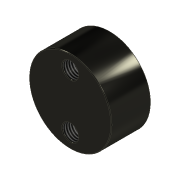
# Autodesk Inventor part: draaischijf HMI
Saved by Autodesk Inventor 2020.3 (Build 243373000, 373)
## iProperties
Created: 2020-12-03
Part Number: draaischijf HMI
Material: Stainless Steel
Document SubType Name: Modeling
Designer: Svend
Density: 8 g/cm^3
Appearance: Gunmetal
Author: Svend
Autodesk Inventor part; units mm, degrees
ref_plane "YZ Plane" through (0, 0, 0) normal (1, 0, 0) x (0, 1, 0)
ref_plane "XZ Plane" through (0, 0, 0) normal (0, 1, 0) x (-1, 0, 0)
ref_plane "XY Plane" through (0, 0, 0) normal (0, 0, 1) x (1, 0, 0)
sketch "Sketch1" plane through (0, 0, 0) normal (0, 0, 1) x (1, 0, 0)
  circle A0 centre (0, 0) radius 13
  circle A1 centre (0, 8.5) radius 2.5
  circle A2 centre (0, -8.5) radius 2.5
  line L0 (0, 8.5) -> (0, -8.5) construction
  dimension "d0" = 26
  dimension "d1" = 5
  dimension "d2" = 17
  constraints: 3 centre point, 2 coincident, 2 end point, 1 equal radius, 1 midpoint, 1 vertical, 1 vertical alignment
  measures "d0" diameter of A0
  measures "d1" diameter of A1
  measures "d2" distance of L0.start L0.end
extrude "Extrusion1" add sketch "Sketch1" along normal blind 12.5
thread "Thread1" size "M5x0.8" class "6H" standard "ANSI Metric M Profile" full length
thread "Thread2" size "M5x0.8" class "6H" standard "ANSI Metric M Profile" full length
fillet "Fillet1" radius 0.2 6 edges at (-13, 0, 12.5) (-13, 0, 0) (-2.5, 8.5, 12.5) (-2.5, -8.5, 12.5) (-2.5, 8.5, 0) (-2.5, -8.5, 0)
body "Solid1"
